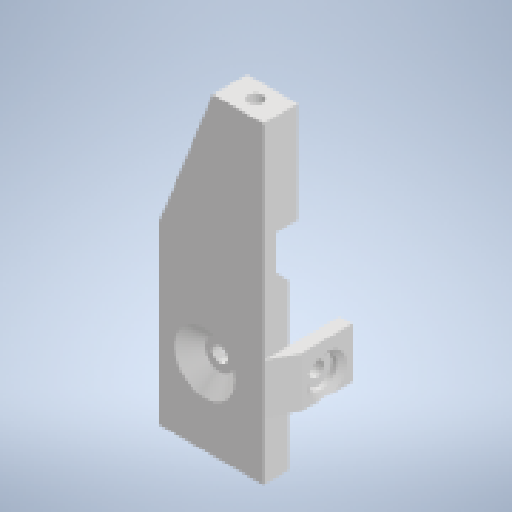
# Autodesk Inventor part: suporte_esquerdo
Saved by Autodesk Inventor 2025.1 (Build 291241000, 241)
## iProperties
Created: 2024-06-30
Part Number: suporte_esquerdo
Material: Genérico
Document SubType Name: Modeling
Designer: joaov
Density: 1 g/cm^3
Appearance: Padrão
Author: joaov
Autodesk Inventor part; units mm, degrees
note: some values were not read from the file. Chosen so that the rebuilt part matches the saved one: second side of "Extrusão11".
ref_plane "YZ Plane" through (0, 0, 0) normal (1, 0, 0) x (0, 1, 0)
ref_plane "XZ Plane" through (0, 0, 0) normal (0, 1, 0) x (-1, 0, 0)
ref_plane "XY Plane" through (0, 0, 0) normal (0, 0, 1) x (1, 0, 0)
sketch "Esboço1" plane through (0, 0, 0) normal (0, 0, 1) x (1, 0, 0)
  line L0 (80.2817, -126.5075) -> (80.2817, -137.9075)
  line L1 (80.2817, -137.9075) -> (59.6627, -137.9075)
  line L2 (77.7817, -126.5075) -> (80.2817, -126.5075)
  line L3 (77.7817, -119.0075) -> (77.7817, -126.5075)
  line L4 (59.6627, -137.9075) -> (59.6627, -102.6075)
  line L5 (80.2817, -116.5075) -> (77.7817, -119.0075)
  line L6 (59.6627, -102.6075) -> (80.2817, -102.6075)
  line L7 (80.2817, -105.1075) -> (80.2817, -116.5075)
  line L8 (80.2817, -102.6075) -> (80.2817, -105.1075)
  line L9 (77.7817, -122.7575) -> (59.6627, -122.7575)
  circle A0 centre (68.7222, -122.7575) radius 1.45
  point P0 (0, 0)
  dimension "d65" = 2.9
  constraints: 20 end point, 4 perpendicular, 2 midpoint, 1 centre point, 1 parallel, 1 point on line
  measures "d65" diameter of A0
extrude "Extrusão1" add sketch "Esboço1" along normal blind 5 contours L0 L1 L4 L9 A0 L3 L2 | L9 A0 L4 L6 L8 L7 L5 L3
sketch "Esboço2" plane through (0, 0, 5) normal (0, 0, 1) x (1, 0, 0)
  line L0 (69.9722, -137.7075) -> (80.6667, -137.7075)
  line L1 (80.6667, -137.7075) -> (80.6667, -138.3178)
  line L2 (80.6667, -138.3178) -> (69.9722, -138.3178)
  line L3 (69.9722, -137.7075) -> (59.8627, -137.7075)
  line L4 (59.358, -137.7075) -> (59.358, -138.3178)
  line L5 (59.358, -138.3178) -> (69.9722, -138.3178)
  line L6 (69.9722, -102.8075) -> (80.6667, -102.8075)
  line L7 (80.6667, -102.8075) -> (80.6667, -102.3974)
  line L8 (80.6667, -102.3974) -> (69.9722, -102.3974)
  line L9 (69.9722, -102.8075) -> (59.8627, -102.8075)
  line L10 (59.358, -102.8075) -> (59.358, -102.3974)
  line L11 (59.358, -102.3974) -> (69.9722, -102.3974)
  line L12 (59.358, -102.6075) -> (59.358, -138.3178)
  line L13 (59.358, -138.3178) -> (59.8627, -138.3178)
  line L14 (59.8627, -137.7075) -> (59.8627, -102.8075)
  point P0 (0, 0)
  constraints: 30 end point, 5 parallel, 4 horizontal, 4 perpendicular
extrude "Extrusão2" cut sketch "Esboço2" against normal through all
sketch "Esboço3" plane through (80.2817, -116.5075, 5) normal (1, 0, 0) x (0, 0, -1)
  line L0 (5, 0) -> (5, 13.7) projected
  line L1 (5, 13.7) -> (2.5, 13.7)
  line L2 (5, 13.7) -> (0, 13.7) projected
  line L3 (5, 13.7) -> (5, 11.2)
  line L4 (2.5, 13.7) -> (5, 11.2)
  point P0 (5, 116.5075)
  dimension "d15" = 2.5
  dimension "d16" = 2.5
  constraints: 6 end point, 1 midpoint, 1 point on line
  measures "d15" distance of L0.end L1.end
  measures "d16" distance of L0.end L3.end
extrude "Extrusão3" cut sketch "Esboço3" against normal through all
sketch "Esboço4" plane through (0, 0, 0) normal (0, 0, -1) x (-1, 0, 0)
  line L0 (-77.7817, -119.0075) -> (-80.2817, -116.5075) projected
  line L1 (-77.7817, -126.5075) -> (-77.7817, -119.0075) projected
  line L2 (-80.2817, -116.5075) -> (-77.7817, -119.0075)
  line L3 (-77.7817, -119.0075) -> (-77.7817, -126.5075)
  line L4 (-77.7817, -126.5075) -> (-80.2817, -126.5075)
  line L5 (-80.2817, -126.5075) -> (-80.2817, -116.5075)
  point P0 (0, 0)
  constraints: 8 end point, 2 perpendicular, 1 collinear
extrude "Extrusão4" add sketch "Esboço4" along normal blind 10
sketch "Esboço5" plane through (0, 0, -10) normal (0, 0, -1) x (-1, 0, 0)
  line L0 (-77.7817, -119.0075) -> (-80.2817, -116.5075) projected
  line L1 (-80.2817, -116.5075) -> (-80.2817, -116.6075)
  line L2 (-80.2817, -116.6075) -> (-77.7817, -119.1075)
  line L3 (-80.2817, -116.5075) -> (-80.2817, -126.5075) projected
  line L4 (-80.2817, -116.5075) -> (-80.2817, -116.1602)
  line L5 (-80.2817, -116.5075) -> (-80.2817, -105.3075) projected
  line L6 (-80.2817, -116.1602) -> (-77.7817, -116.1602)
  line L7 (-77.7817, -116.1602) -> (-77.7817, -119.1075)
  line L8 (-80.2817, -126.5075) -> (-80.2817, -126.4075)
  line L9 (-80.2817, -126.4075) -> (-77.6383, -126.4075)
  line L10 (-77.6383, -126.4075) -> (-77.6383, -126.5963)
  line L11 (-77.6383, -126.5963) -> (-80.2817, -126.5963)
  line L12 (-80.2817, -126.5963) -> (-80.2817, -126.4075)
  point P0 (0, 0)
  dimension "d26" = 0.1
  constraints: 20 end point, 2 horizontal, 2 parallel, 2 perpendicular, 2 point on line
  measures "d26" distance of L3.end L8.end
extrude "Extrusão5" cut sketch "Esboço5" against normal blind 10 contours L0 L4 L6 L7 | L9 L10 L11 L12 L3
sketch "Esboço6" plane through (0, 0, 5) normal (0, 0, 1) x (1, 0, 0)
  line L0 (80.2817, -126.5075) -> (77.7817, -126.5075) projected
  line L1 (80.2817, -126.5075) -> (77.7817, -126.5075)
  line L2 (77.7817, -119.0075) -> (80.2817, -116.5075) projected
  line L3 (77.7817, -126.5075) -> (77.7817, -119.0075)
  line L4 (77.7817, -119.0075) -> (80.2817, -116.5075)
  line L5 (80.2817, -116.5075) -> (80.2817, -126.5075)
  point P0 (0, 0)
  constraints: 8 end point, 1 collinear, 1 horizontal, 1 parallel, 1 perpendicular
extrude "Extrusão6" add sketch "Esboço6" against normal blind 5
sketch "Esboço7" plane through (80.2817, -137.7075, 5) normal (1, 0, 0) x (0, 0, -1)
  line L0 (5, 21.2) -> (15, 21.2) projected
  line L1 (15, 21.2) -> (15, 18.7)
  line L2 (15, 21.2) -> (15, 11.3) projected
  line L3 (5, 18.7) -> (5, 21.2) projected
  line L4 (15, 18.7) -> (5, 18.7)
  line L5 (5, 18.7) -> (5, 21.2)
  line L6 (5, 21.2) -> (15, 21.2)
  line L7 (15, 11.3) -> (5, 11.3) projected
  line L8 (5, 11.3) -> (15, 18.7)
  circle A0 centre (10, 15) radius 1.45
  point P0 (5, 137.7075)
  dimension "d31" = 2.5
  dimension "d32" = 2.9
  constraints: 10 end point, 1 centre point, 1 collinear, 1 midpoint, 1 perpendicular, 1 point on line
  measures "d31" distance of L0.end L1.end
  measures "d32" diameter of A0
extrude "Extrusão7" cut sketch "Esboço7" against normal blind 5 contours A0 L8 | L8 A0
sketch "Esboço8" plane through (0, 0, 5) normal (0, 0, 1) x (1, 0, 0)
  line L0 (80.2817, -137.7075) -> (80.2817, -102.8075) projected
  line L1 (80.2817, -102.8075) -> (80.2817, -95.9075)
  line L2 (80.2817, -95.9075) -> (50.2817, -95.9075)
  line L3 (50.2817, -95.9075) -> (50.2817, -102.8075)
  line L4 (80.2817, -102.8075) -> (59.8627, -102.8075) projected
  line L5 (50.2817, -102.8075) -> (80.2817, -102.8075)
  point P0 (0, 0)
  dimension "d35" = 6.9
  dimension "d36" = 30
  constraints: 8 end point, 2 perpendicular, 1 collinear, 1 vertical
  measures "d35" distance of L0.end L1.end
  measures "d36" distance of L1.end L2.end
extrude "Extrusão8" add sketch "Esboço8" against normal blind 2.5
sketch "Esboço10" plane through (50.2817, -95.9075, 5) normal (0, 1, 0) x (1, 0, 0)
  line L0 (30, 0) -> (30, 2.5) projected
  line L1 (30, 5) -> (30, 2.5) projected
  line L2 (30, 0) -> (30, 2.5)
  line L3 (30, 2.5) -> (30, 6.8)
  line L4 (30, 6.8) -> (0, 6.8)
  line L5 (0, 0) -> (0, 2.5) projected
  line L6 (0, 6.8) -> (0, 0)
  line L7 (0, 0) -> (30, 0)
  point P0 (-50.2817, 5)
  dimension "d39" = 4.3
  constraints: 10 end point, 3 perpendicular, 1 point on line, 1 vertical
  measures "d39" distance of L0.end L3.end
extrude "Extrusão9" add sketch "Esboço10" along normal blind 2.5
sketch "Esboço11" plane through (50.2817, -93.4075, 5) normal (0, 1, 0) x (1, 0, 0)
  line L0 (30, 2.5) -> (30, 6.8) projected
  line L1 (30, 5) -> (30, 2.5) projected
  line L2 (30, 6.8) -> (30, 2.5)
  line L3 (0, 0) -> (0, 2.5) projected
  line L4 (30, 2.5) -> (0, 2.5)
  line L5 (0, 6.8) -> (0, 2.5) projected
  line L6 (0, 2.5) -> (0, 6.8)
  line L7 (0, 6.8) -> (30, 6.8)
  line L8 (0, 2.5) -> (30, 2.5)
  line L9 (30, 2.5) -> (30, 0)
  line L10 (30, 0) -> (0, 0)
  line L11 (0, 0) -> (0, 2.5)
  point P0 (-50.2817, 5)
  dimension "d42" = 4.3
  constraints: 16 end point, 4 perpendicular, 2 parallel, 1 collinear, 1 horizontal
  measures "d42" distance of L0.end L0.start
extrude "Extrusão10" add sketch "Esboço11" along normal blind 12.3
sketch "Esboço12" plane through (80.2817, -95.9075, -1.8) normal (0, 0, -1) x (-1, 0, 0)
  line L0 (0, 14.8) -> (30, 14.8) projected
  line L1 (0, 14.8) -> (30, 14.8)
  line L2 (30, 14.8) -> (30, 19.8)
  line L3 (30, 19.8) -> (0, 19.8)
  line L4 (0, 19.8) -> (0, 14.8)
  point P0 (80.2817, 95.9075)
  dimension "d45" = 5
  constraints: 8 end point, 2 parallel, 1 horizontal, 1 perpendicular
  measures "d45" distance of L2.end L1.end
extrude "Extrusão11" add sketch "Esboço12" against normal blind 6.8
sketch "Esboço14" plane through (80.2817, -137.7075, 5) normal (1, 0, 0) x (0, 0, -1)
  line L0 (5, 18.7) -> (5, 21.2) projected
  line L1 (15, 21.2) -> (15, 11.3) projected
  line L2 (5, 21.2) -> (15, 21.2)
  line L3 (15, 21.2) -> (15, 11.3)
  line L4 (15, 11.3) -> (5, 11.3)
  line L5 (5, 11.3) -> (5, 21.2)
  circle A0 centre (10, 15) radius 1.45 projected
  circle A1 centre (10, 15) radius 1.45
  point P0 (5, 137.7075)
  constraints: 8 end point, 2 parallel, 1 centre point, 1 coincident, 1 horizontal, 1 perpendicular
extrude "Extrusão13" add sketch "Esboço14" along normal blind 2.5
sketch "Esboço15" plane through (77.7817, -126.4075, -10) normal (0, -1, 0) x (1, 0, 0)
  line L0 (5, 10) -> (5, 0) projected
  line L1 (2.5, 15) -> (2.5, 10) projected
  line L2 (5, 10) -> (2.5, 10)
  line L3 (2.5, 10) -> (2.5, 15)
  line L4 (2.5, 15) -> (5, 10)
  point P0 (-77.7817, 10)
  constraints: 6 end point, 1 horizontal, 1 perpendicular
extrude "Extrusão14" add sketch "Esboço15" against normal blind 9.9
sketch "Esboço16" plane through (50.2817, -76.1075, -1.8) normal (0, 1, 0) x (1, 0, 0)
  line L0 (30, 0) -> (0, 0) projected
  line L1 (15, 0) -> (15, -6.8)
  line L2 (9.581, -6.8) -> (30, -6.8) projected
  line L3 (15, -3.4) -> (30, -3.4)
  line L4 (30, -3.4) -> (25, -3.4)
  circle A0 centre (25, -3.4) radius 1.4
  point P0 (-50.2817, -1.8)
  dimension "d92" = 5
  dimension "d99" = 2.8
  constraints: 6 end point, 2 midpoint, 2 point on line, 1 centre point, 1 horizontal, 1 vertical
  measures "d92" distance of L3.end L4.end
  measures "d99" diameter of A0
extrude "Extrusão15" cut sketch "Esboço16" against normal blind 10
sketch "Esboço18" plane through (0, 0, 5) normal (0, 0, 1) x (1, 0, 0)
  line L0 (80.2817, -116.5075) -> (80.2817, -76.1075) projected
  line L1 (80.2817, -76.1075) -> (70.2817, -76.1075)
  line L2 (50.2817, -76.1075) -> (80.2817, -76.1075) projected
  line L3 (80.2817, -102.8075) -> (59.8627, -102.8075) projected
  line L4 (70.2817, -76.1075) -> (59.8627, -102.8075)
  line L5 (59.8627, -102.8075) -> (80.2817, -102.8075)
  line L6 (80.2817, -102.8075) -> (80.2817, -76.1075)
  line L7 (70.2817, -76.1075) -> (50.2817, -76.1075)
  line L8 (50.2817, -76.1075) -> (50.2817, -102.8075) projected
  line L9 (50.2817, -102.8075) -> (59.8627, -102.8075)
  line L10 (50.2817, -102.8075) -> (50.2817, -76.1075)
  point P0 (0, 0)
  dimension "d96" = 10
  constraints: 14 end point, 2 perpendicular, 1 collinear, 1 horizontal, 1 parallel, 1 point on line
  measures "d96" distance of L0.end L1.end
extrude "Extrusão16" cut sketch "Esboço18" against normal through all contours L9 L8 L2 L4
sketch "Esboço19" plane through (0, 0, 5) normal (0, 0, 1) x (1, 0, 0)
  circle A0 centre (68.7222, -122.7575) radius 1.45 projected
  circle A1 centre (68.7222, -122.7575) radius 1.45
  circle A2 centre (68.7222, -122.7575) radius 2.95
  point P0 (0, 0)
  dimension "d100" = 5.9
  constraints: 2 centre point, 2 coincident
  measures "d100" diameter of A2
extrude "Extrusão17" cut sketch "Esboço19" against normal blind 3
chamfer "Chanfro9" distance 3 angle 45 1 edges at (65.7722, -122.7575, 5)
sketch "Esboço20" plane through (82.7817, -137.7075, 5) normal (1, 0, 0) x (0, 0, -1)
  circle A0 centre (10, 15) radius 1.45 projected
  circle A1 centre (10, 15) radius 1.45
  circle A2 centre (10, 15) radius 2.95
  point P0 (5, 137.7075)
  dimension "d106" = 5.9
  constraints: 2 centre point, 2 coincident
  measures "d106" diameter of A2
extrude "Extrusão18" cut sketch "Esboço20" against normal blind 2
chamfer "Chanfro10" distance 1 angle 45 1 edges at (82.7817, -122.7075, -2.05)
